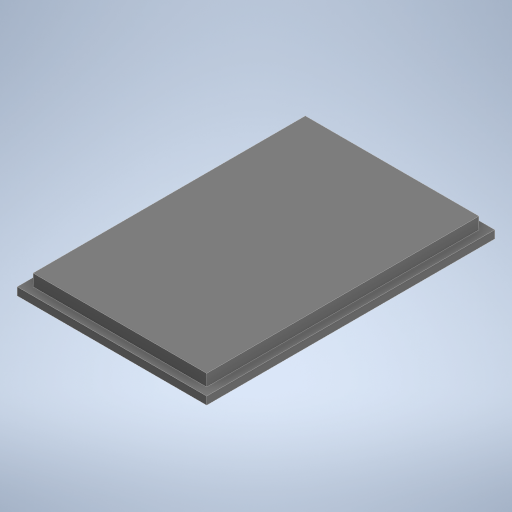
# Autodesk Inventor part: LCD
Saved by Autodesk Inventor 2023 (Build 270158000, 158)
## iProperties
Created: 2022-11-17
Part Number: LCD
Material: Generic
Document SubType Name: Modeling
Designer: spfow
Density: 1 g/cm^3
Appearance: Gray
Author: spfow
Autodesk Inventor part; units mm, degrees
ref_plane "YZ Plane" through (0, 0, 0) normal (1, 0, 0) x (0, 1, 0)
ref_plane "XZ Plane" through (0, 0, 0) normal (0, 1, 0) x (-1, 0, 0)
ref_plane "XY Plane" through (0, 0, 0) normal (0, 0, 1) x (1, 0, 0)
sketch "Sketch1" plane through (0, 0, 0) normal (0, 1, 0) x (-1, 0, 0)
  line L0 (0, 0) -> (55.88, 0)
  line L1 (55.88, 0) -> (55.88, -87.63)
  line L2 (55.88, -87.63) -> (0, -87.63)
  line L3 (0, -87.63) -> (0, 0)
  line L4 (58.42, -90.17) -> (58.42, 2.54)
  line L5 (58.42, 2.54) -> (-2.54, 2.54)
  line L6 (-2.54, 2.54) -> (-2.54, -90.17)
  line L7 (-2.54, -90.17) -> (58.42, -90.17)
  dimension "d0" = 55.88
  dimension "d1" = 87.63
  dimension "d2" = 2.54
  constraints: 16 end point, 4 parallel, 2 perpendicular, 1 horizontal, 3 other
  measures "d0" distance of L1.end L2.end
  measures "d1" distance of L0.end L1.end
  measures "d2" distance between parallel lines of L1 L4
extrude "Extrusion1" add sketch "Sketch1" along normal blind 6.35 contours L0 L1 L2 L3
extrude "Extrusion2" add sketch "Sketch1" along normal blind 2.54
body "Solid1"
